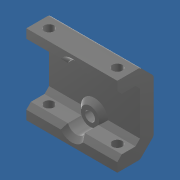
# Autodesk Inventor part: X_End_Holder
Saved by Autodesk Inventor 2020 (Build 240168000, 168)
## iProperties
Created: 2021-05-10
Part Number: X_End_Holder
Material: 一般
Document SubType Name: Modeling
Designer: ken113
Density: 1 g/cm^3
Appearance: 滑らか - 黒
Author: ken113
Autodesk Inventor part; units mm, degrees
ref_plane "YZ Plane" through (0, 0, 0) normal (1, 0, 0) x (0, 1, 0)
ref_plane "XZ Plane" through (0, 0, 0) normal (0, 1, 0) x (-1, 0, 0)
ref_plane "XY Plane" through (0, 0, 0) normal (0, 0, 1) x (1, 0, 0)
sketch "スケッチ1" plane through (0, 0, 0) normal (0, 0, 1) x (1, 0, 0)
  line L0 (20, -17.5) -> (-20, -17.5)
  line L1 (-20, -17.5) -> (-20, 17.5)
  line L2 (-20, 17.5) -> (20, 17.5)
  line L3 (20, 17.5) -> (20, -17.5)
  line L4 (20, -17.5) -> (-20, 17.5) construction
  line L5 (-20, -17.5) -> (20, 17.5) construction
  point P0 (0, 0)
  dimension "d0" = 35
  dimension "d1" = 40
  constraints: 12 end point, 2 midpoint, 2 parallel, 1 horizontal, 1 perpendicular
  measures "d0" distance of L2.end L0.start
  measures "d1" distance of L1.end L2.end
extrude "押し出し1" add sketch "スケッチ1" along normal blind 6
sketch "スケッチ2" plane through (0, 0, 6) normal (0, 0, 1) x (1, 0, 0)
  line L0 (-20, -17.5) -> (20, -17.5) projected
  line L1 (20, -17.5) -> (20, 17.5) projected
  line L2 (-20, -17.5) -> (20, -17.5)
  line L3 (20, -17.5) -> (20, -11.5)
  line L4 (20, -11.5) -> (-20, -11.5)
  line L5 (-20, -11.5) -> (-20, -17.5)
  line L6 (-20, 17.5) -> (-20, -17.5) projected
  line L7 (20, 17.5) -> (-20, 17.5)
  line L8 (-20, 17.5) -> (-20, 11.5)
  line L9 (-20, 11.5) -> (20, 11.5)
  line L10 (20, 11.5) -> (20, 17.5)
  point P0 (0, 0)
  point P1 (20, 11.5)
  dimension "d4" = 6
  dimension "d5" = 6
  constraints: 16 end point, 4 parallel, 2 horizontal, 2 perpendicular, 2 point on line
  measures "d4" distance between parallel lines of L7 L9
  measures "d5" distance between parallel lines of L4 L0
extrude "押し出し2" add sketch "スケッチ2" along normal blind 10 contours L5 L4 L1 L0 | L6 L7 L1 L9
sketch "スケッチ3" plane through (-20, -17.5, 0) normal (0, -1, 0) x (1, 0, 0)
  line L0 (0, 0) -> (40, 0) projected
  line L1 (40, 0) -> (40, 16) projected
  line L2 (0, 16) -> (40, 16) projected
  line L3 (0, 0) -> (0, 16) projected
  point P0 (20, 0)
  point P1 (5, 11)
  point P2 (35, 11)
  dimension "d8" = 30
  dimension "d9" = 5
  dimension "d10" = 15
  constraints: 1 horizontal alignment
  measures "d8" distance of point (35, 11) point (5, 11)
  measures "d9" distance from line of point (35, 11) L2
  measures "d10" horizontal distance of point (5, 11) point (20, 0)
hole "穴1" at (-15, -17.5, 11) at (15, -17.5, 11) direction (0, 1, 0) diameter 4.4 end through all
sketch "スケッチ4" plane through (0, 0, 6) normal (0, 0, 1) x (1, 0, 0)
  line L0 (-20, -11.5) -> (20, -11.5) projected
  line L1 (20, -11.5) -> (20, 11.5) projected
  line L2 (20, 11.5) -> (-20, 11.5) projected
  line L3 (-20, 11.5) -> (-20, -11.5) projected
  line L4 (0, 10) -> (0, -10) construction
  line L5 (-4, 10) -> (-4, -10)
  line L6 (4, -10) -> (4, 10)
  arc A0 (4, 10) -> (-4, 10) centre (0, 10) ccw
  arc A1 (-4, -10) -> (4, -10) centre (0, -10) ccw
  point P0 (0, 0)
  point P1 (0, 0)
  dimension "d18" = 20
  dimension "d19" = 4
  dimension "d20" = 0
  constraints: 8 end point, 4 point on circle, 4 tangent, 2 centre point, 1 midpoint, 1 parallel, 1 vertical
  measures "d18" distance of L4.start L4.end
  measures "d19" radius of A1
  measures "d20" distance from line of L4 point (0, 0)
extrude "押し出し3" cut sketch "スケッチ4" along normal blind 10 contours A1 L5 A0 L2 L6 L0 | L0 A1 | A0 L2
sketch "スケッチ5" plane through (0, 0, 6) normal (0, 0, 1) x (1, 0, 0)
  line L0 (-3.7081, 11.5) -> (-20, 11.5) projected
  line L1 (-20, 11.5) -> (-20, -11.5) projected
  line L2 (-20, -11.5) -> (-3.7081, -11.5) projected
  arc A0 (-3.7081, -11.5) -> (3.7081, -11.5) centre (0, -10) ccw projected
  line L3 (3.7081, -11.5) -> (20, -11.5) projected
  line L4 (20, -11.5) -> (20, 11.5) projected
  line L5 (20, 11.5) -> (3.7081, 11.5) projected
  arc A1 (3.7081, 11.5) -> (-3.7081, 11.5) centre (0, 10) ccw projected
  circle A2 centre (0, -10) radius 4
  circle A3 centre (0, 10) radius 4
  point P0 (0, 0)
  point P1 (3.7081, 11.5)
  constraints: 2 coincident, 1 centre point, 1 concentric, 3 other
extrude "押し出し4" add sketch "スケッチ5" along normal blind 2 contours A1 A3 | A2 A0
sketch "スケッチ6" plane through (0, 0, 8) normal (0, 0, 1) x (1, 0, 0)
  arc A0 (3.7081, 11.5) -> (-3.7081, 11.5) centre (0, 10) ccw projected
  arc A1 (-3.7081, 11.5) -> (3.7081, 11.5) centre (0, 10) ccw projected
  arc A2 (-3.7081, -11.5) -> (3.7081, -11.5) centre (0, -10) ccw projected
  arc A3 (3.7081, -11.5) -> (-3.7081, -11.5) centre (0, -10) ccw projected
  point P0 (0, 0)
hole "穴2" at (0, -10, 8) at (0, 10, 8) direction (0, 0, -1) diameter 4.4 depth 6
chamfer "面取り1" distance 2 angle 45 6 edges at (0, 6, 6) (0, -6, 6) (-11.854, -11.5, 6) (11.854, -11.5, 6) (11.854, 11.5, 6) (-11.854, 11.5, 6)
chamfer "面取り2" distance 6 angle 45 2 edges at (0, 17.5, 0) (0, -17.5, 0)
chamfer "面取り3" distance 2 angle 45 6 edges at (11.854, -11.5, 16) (0, -14, 16) (-11.854, -11.5, 16) (-11.854, 11.5, 16) (0, 14, 16) (11.854, 11.5, 16)
fillet "フィレット1" radius 2 4 edges at (0, 17.5, 6) (0, 11.5, 0) (0, -11.5, 0) (0, -17.5, 6)
equation "\"d4\" = d5"
